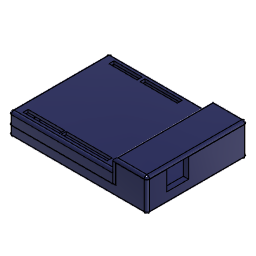
Arduino Case (Autodesk Fusion 360 design; units mm, degrees)
Autodesk Fusion 360 part; units mm, degrees
sketch "Footprint" plane through (0, 0, 0) normal (0, 0, 1) x (1, 0, 0) in component "Box"
  line L0 (-37.3689, 24.9646) -> (33.9311, 24.9646)
  line L1 (33.9311, 24.9646) -> (33.9311, -28.6454)
  line L2 (33.9311, -28.6454) -> (-37.3689, -28.6454)
  line L3 (-39.9289, -28.6454) -> (-39.9289, 24.9646) construction
  line L4 (-37.3689, 24.9646) -> (-37.3689, 23.8242)
  line L5 (-37.3689, -17.1454) -> (-37.3689, -28.6454)
  line L6 (-39.9289, -12.7954) -> (-39.9289, 20.8146)
  line L7 (-37.3689, -28.6454) -> (-39.9289, -28.6454) construction
  line L8 (-37.3689, 24.9646) -> (-39.9289, 24.9646) construction
  spline S0 degree 5 poles (-37.3689, -17.1454) (-37.4677, -17.1053) (-37.6612, -17.0209) (-37.9387, -16.8819) (-38.2829, -16.671) (-38.6672, -16.3623) (-39.0017, -16.0045) (-39.2827, -15.5942) (-39.5091, -15.13) (-39.6839, -14.6151) (-39.8112, -14.0534) (-39.8784, -13.57) (-39.9106, -13.1896) (-39.9241, -12.9281) (-39.9289, -12.7954) knots 0 0 0 0 0 0 0.1 0.2 0.3 0.4 0.5 0.6 0.7 0.8 0.9 1 1 1 1 1 1
  spline S1 degree 5 poles (-37.3689, 23.8242) (-37.4546, 23.8427) (-37.6228, 23.8724) (-37.8658, 23.8956) (-38.1706, 23.8828) (-38.5177, 23.7895) (-38.8283, 23.6128) (-39.1, 23.3478) (-39.3331, 22.9945) (-39.5301, 22.5591) (-39.6944, 22.0491) (-39.802, 21.5868) (-39.8702, 21.2116) (-39.9102, 20.949) (-39.9289, 20.8146) knots 0 0 0 0 0 0 0.1 0.2 0.3 0.4 0.5 0.6 0.7 0.8 0.9 1 1 1 1 1 1
  circle A0 centre (-37.3739, -10.6904) radius 1.395
  circle A1 centre (-37.3739, 17.3996) radius 1.395
  circle A2 centre (14.9261, 22.4096) radius 1.395
  circle A3 centre (13.6061, -26.0904) radius 1.395
  line L9 (33.9311, 24.9646) -> (36.9311, 24.9646)
  line L10 (36.9311, 24.9646) -> (36.9311, -28.6454)
  line L11 (36.9311, -28.6454) -> (33.9311, -28.6454)
  line L12 (36.9311, 24.9646) -> (36.9311, 26.7646)
  line L13 (36.9311, 26.7646) -> (-41.7289, 26.7646)
  line L14 (-41.7289, 26.7646) -> (-41.7289, -30.4454)
  line L15 (-41.7289, -30.4454) -> (36.9311, -30.4454)
  line L16 (36.9311, -30.4454) -> (36.9311, -28.6454)
  line L17 (33.9311, -19.1004) -> (36.9311, -19.1004)
  line L18 (36.9311, -6.6204) -> (33.9311, -6.6204)
  line L19 (19.2711, -30.4454) -> (19.2711, -28.6454)
  line L20 (19.2711, 24.9646) -> (19.2711, 26.7646)
  point P0 (-39.2184, -15.6652)
  point P1 (-38.9763, 23.4524)
  dimension "d4" = 53.61
  dimension "d6" = 73.86
  dimension "d8" = 2.56
  dimension "d10" = 33.61
  dimension "d12" = 15.85
  dimension "d14" = 2.79
  dimension "d15" = 17.955
  dimension "d16" = 2.555
  dimension "d17" = 7.565
  dimension "d18" = 2.555
  dimension "d19" = 2.555
  dimension "d20" = 20.325
  dimension "d21" = 19.005
  dimension "d22" = 3
  dimension "d23" = 1.8
  dimension "d24" = 1.8
  dimension "d25" = 1.8
  dimension "d31" = 9.545
  dimension "d32" = 12.48
  dimension "d38" = 14.66
  dimension "d47" = 11.5
  constraint horizontal L0
  constraint vertical L1
  constraint horizontal L2
  constraint vertical L3
  constraint perpendicular L0 L4
  constraint coincident L3 L6.end
  constraint coincident L3 L6.start
  constraint perpendicular L2 L5
  constraint collinear L4 L5
  constraint perpendicular L3 L7
  constraint perpendicular L3 L8
  constraint equal A0 A1
  constraint vertical A0.centre A1.centre
  constraint equal A0 A3
  constraint equal A0 A2
  constraint perpendicular L1 L9
  constraint perpendicular L2 L10
  constraint perpendicular L1 L11
  constraint perpendicular L9 L12
  constraint perpendicular L12 L13
  constraint perpendicular L13 L14
  constraint perpendicular L10 L15
  constraint perpendicular L11 L16
  constraint coincident L1 L17.start
  constraint coincident L10 L17.end
  constraint perpendicular L10 L17
  constraint coincident L10 L18.start
  constraint coincident L1 L18.end
  constraint perpendicular L1 L18
  constraint coincident L15 L19.start
  constraint coincident L2 L19.end
  constraint perpendicular L2 L19
  constraint coincident L0 L20.start
  constraint coincident L13 L20.end
  constraint perpendicular L13 L20
  constraint collinear L19 L20
  measures "d4" distance of L0 L2
  measures "d6" distance of L1 L3
  measures "d8" distance of L3 L5
  measures "d10" distance of L6.end L6.start
  measures "d12" distance of L2 L6.start
  measures "d14" diameter of A0
  measures "d15" distance of L2 A0.centre
  measures "d16" distance of L3 A0.centre
  measures "d17" distance of L0 A1.centre
  measures "d18" distance of L2 A3.centre
  measures "d19" distance of L0 A2.centre
  measures "d20" distance of L1 A3.centre
  measures "d21" distance of L1 A2.centre
  measures "d22" distance of L1 L10
  measures "d23" distance of L0 L13
  measures "d24" distance of L2 L15
  measures "d25" distance of L6 L14
  measures "d31" distance of L2 L17
  measures "d32" distance of L17 L18
  measures "d38" distance of L1 L19
  measures "d47" distance of L5.start L2.end
extrude "Extrude1" add sketch "Footprint" along normal blind 1.8 contours L0 L2 L4 L5 L6 S0 S1 L13 L14 L15 L19 L20 | L0 L1 L2 L4 L5 L6 S0 S1 | L0 L9 L12 L13 L20 | L1 L9 L10 L18 | L1 L10 L17 L18 | L1 L10 L11 L17 | L2 L11 L15 L16 L19 | A0 | A1 | A2 | A3 makes body 1 in component "Box"
extrude "Extrude2" add sketch "Footprint" along normal blind 4.5 from surface at 1.8 contours L0 L2 L4 L5 L6 S0 S1 L13 L14 L15 L19 L20 | L0 L9 L12 L13 L20 | L1 L9 L10 L18 | L1 L10 L17 L18 | L1 L10 L11 L17 | L2 L11 L15 L16 L19 | A0 | A1 | A2 | A3 bodies 1 in component "Box"
extrude "Extrude3" add sketch "Footprint" along normal blind 11.08 from surface at 6.3 contours L0 L9 L12 L13 L20 | L1 L9 L10 L18 | L1 L10 L11 L17 | L2 L11 L15 L16 L19 bodies 1 in component "Box"
sketch "Side Profile" plane through (0, 26.7646, 0) normal (0, 1, 0) x (-1, 0, 0) in component "FrontCover"
  line L0 (-19.2711, 6.3) -> (-19.2711, 17.38) construction
  line L1 (-36.9311, 17.38) -> (-19.2711, 17.38) construction
  line L2 (-36.9311, 17.535) -> (-19.1161, 17.535)
  line L3 (-19.1161, 17.535) -> (-19.1161, 6.455)
  line L4 (-19.1161, 6.455) -> (-17.5161, 6.455)
  line L5 (-17.5161, 6.455) -> (-17.5161, 19.035)
  line L6 (-17.5161, 19.035) -> (-36.9311, 19.035)
  line L7 (-36.9311, 19.035) -> (-36.9311, 17.535)
  dimension "d39" = 0.155
  dimension "d40" = 0.155
  dimension "d44" = 0.155
  dimension "d45" = 1.5
  dimension "d46" = 1.6
  constraint parallel L1 L2
  constraint perpendicular L2 L3
  constraint perpendicular L3 L4
  constraint perpendicular L4 L5
  constraint perpendicular L5 L6
  constraint perpendicular L2 L7
  constraint collinear L1.start L2.start L6.end
  measures "d39" distance of L1 L2
  measures "d40" distance of L0 L3
  measures "d44" distance of L0.start L4
  measures "d45" distance of L2 L6
  measures "d46" distance of L3 L5
extrude "Extrude1'" add sketch "Side Profile" against normal up to surface (57.21 mm away) separate body makes body 2 in component "FrontCover"
ref_plane "WorkPlane1" through (-11.2289, -1.8404, 11.4) normal (0, 0, 1) x (1, 0, 0) in component "Lid"
sketch "Footprint (2)" plane through (0, 0, 11.4) normal (0, 0, 1) x (-1, 0, 0) in component "Lid"
  line L0 (-33.9311, 28.6454) -> (37.3689, 28.6454) construction
  line L1 (37.3689, 17.1454) -> (37.3689, 28.6454)
  spline S0 degree 5 poles (37.3689, 17.1454) (37.4677, 17.1053) (37.6612, 17.0209) (37.9387, 16.8819) (38.2829, 16.671) (38.6672, 16.3623) (39.0017, 16.0045) (39.2827, 15.5942) (39.5091, 15.13) (39.6839, 14.6151) (39.8112, 14.0534) (39.8784, 13.57) (39.9106, 13.1896) (39.9241, 12.9281) (39.9289, 12.7954) knots 0 0 0 0 0 0 0.1 0.2 0.3 0.4 0.5 0.6 0.7 0.8 0.9 1 1 1 1 1 1
  line L2 (39.9289, 12.7954) -> (39.9289, -20.8146)
  spline S1 degree 5 poles (37.3689, -23.8242) (37.4546, -23.8427) (37.6228, -23.8724) (37.8658, -23.8956) (38.1706, -23.8828) (38.5177, -23.7895) (38.8283, -23.6128) (39.1, -23.3478) (39.3331, -22.9945) (39.5301, -22.5591) (39.6944, -22.0491) (39.802, -21.5868) (39.8702, -21.2116) (39.9102, -20.949) (39.9289, -20.8146) knots 0 0 0 0 0 0 0.1 0.2 0.3 0.4 0.5 0.6 0.7 0.8 0.9 1 1 1 1 1 1
  line L3 (37.3689, -24.9646) -> (37.3689, -23.8242)
  line L4 (37.3689, -24.9646) -> (-33.9311, -24.9646) construction
  line L5 (41.7289, -26.7646) -> (-17.5161, -26.7646)
  line L6 (-17.5161, -26.7646) -> (-17.5161, -24.9646)
  line L7 (37.3689, -24.9646) -> (-17.5161, -24.9646)
  line L8 (37.3689, 28.6454) -> (-17.5161, 28.6454)
  line L9 (-17.5161, 30.4454) -> (-17.5161, 28.6454)
  line L10 (-17.5161, 30.4454) -> (41.7289, 30.4454)
  line L11 (41.7289, 30.4454) -> (41.7289, -26.7646)
  line L12 (-17.5161, -24.9646) -> (-17.5161, 28.6454)
  line L13 (36.6039, 27.4304) -> (-11.3161, 27.4304)
  line L14 (-11.3161, 27.4304) -> (-11.3161, 24.6204)
  line L15 (-11.3161, 24.6204) -> (36.6039, 24.6204)
  line L16 (36.6039, 24.6204) -> (36.6039, 27.4304)
  line L17 (36.0739, -23.7896) -> (-2.8261, -23.7896)
  line L18 (-2.8261, -23.7896) -> (-2.8261, -20.9796)
  line L19 (-2.8261, -20.9796) -> (36.0739, -20.9796)
  line L20 (36.0739, -20.9796) -> (36.0739, -23.7896)
  line L21 (15.7639, 24.6204) -> (15.7639, 27.4304)
  line L22 (14.8339, 24.6204) -> (14.8339, 27.4304)
  line L23 (20.0439, -23.7896) -> (20.0439, -20.9796)
  line L24 (18.3339, -23.7896) -> (18.3339, -20.9796)
  point P0 (41.7289, -26.7646)
  point P1 (-19.2711, -26.7646)
  point P2 (-19.2711, 30.4454)
  point P3 (41.7289, 30.4454)
  dimension "d48" = 1.755
  dimension "d58" = 0.765
  dimension "d59" = 2.81
  dimension "d60" = 20.84
  dimension "d61" = 0.93
  dimension "d62" = 26.15
  dimension "d63" = 1.215
  dimension "d64" = 1.295
  dimension "d65" = 16.03
  dimension "d66" = 1.71
  dimension "d67" = 21.16
  dimension "d68" = 2.81
  dimension "d69" = 1.175
  constraint coincident P0 L5.start
  constraint horizontal L5
  constraint coincident L4 L6.end
  constraint perpendicular L4 L6
  constraint coincident L3.start L4.start
  constraint coincident L0.end L1.end
  constraint coincident L0 L8.end
  constraint perpendicular L8 L9
  constraint coincident P3 L10.end
  constraint perpendicular L9 L10
  constraint collinear L6 L9
  constraint horizontal L13
  constraint vertical L14
  constraint horizontal L15
  constraint vertical L16
  constraint horizontal L17
  constraint vertical L18
  constraint horizontal L19
  constraint vertical L20
  constraint coincident L15 L21.start
  constraint coincident L13 L21.end
  constraint perpendicular L13 L21
  constraint coincident L15 L22.start
  constraint coincident L13 L22.end
  constraint perpendicular L13 L22
  constraint coincident L17 L23.start
  constraint coincident L19 L23.end
  constraint perpendicular L19 L23
  constraint coincident L17 L24.start
  constraint coincident L19 L24.end
  constraint perpendicular L19 L24
  measures "d48" distance of P1 L6
  measures "d58" distance of L1 L16
  measures "d59" distance of L13 L15
  measures "d60" distance of L16 L21
  measures "d61" distance of L21 L22
  measures "d62" distance of L14 L22
  measures "d63" distance of L8 L13
  measures "d64" distance of S1.start L20
  measures "d65" distance of L20 L23
  measures "d66" distance of L23 L24
  measures "d67" distance of L18 L24
  measures "d68" distance of L17 L19
  measures "d69" distance of L4 L17
extrude "Extrude1''" add sketch "Footprint (2)" along normal blind 1.6 separate body contours L1 S0 L2 S1 L3 L7 L8 L12 | L1 S0 L2 S1 L3 L5 L6 L7 L8 L9 L10 L11 | L13 L15 L21 L22 | L17 L19 L23 L24 makes body 3 in component "Lid"
extrude "Extrude2'" add sketch "Footprint (2)" against normal up to surface (5.255 mm away) contours L1 S0 L2 S1 L3 L5 L6 L7 L8 L9 L10 L11 bodies 3 in component "Lid"
fillet "Fillet1" radius 1.5 4 edges at (-41.7289, 26.7646, 3.15) (36.9311, 26.7646, 8.69) (36.9311, -30.4454, 8.69) (-41.7289, -30.4454, 3.15) 1 faces at (-15.5089, 7.6946, 0) on bodies 1 in component "Box"
fillet "Fillet1'" radius 1.5 6 edges at (27.2236, 26.7646, 19.035) (36.9311, 26.7646, 18.285) (27.2236, -30.4454, 19.035) (36.9311, -30.4454, 18.285) (17.5161, -1.8404, 19.035) (36.9311, -1.8404, 19.035) on bodies 2 in component "FrontCover"
fillet "Fillet1''" radius 1.5 5 edges at (-41.7289, 26.7646, 9.5725) (-41.7289, -30.4454, 9.5725) (-41.7289, -1.8404, 13) (-12.1064, -30.4454, 13) (-12.1064, 26.7646, 13) on bodies 3 in component "Lid"
component "Box" placed x (1, 0, 0) y (0, 1, 0) z (0, 0, 1) at (0, 0, 0)
component "FrontCover" placed x (1, 0, 0) y (0, 1, 0) z (0, 0, 1) at (0, 0, 0)
component "Lid" placed x (1, 0, 0) y (0, 1, 0) z (0, 0, 1) at (0, 0, 0)
equation "Tolerance = 0.17 mm" comment "Tolerance to use when PLA/PETG parts mate with existing parts (like a a screw), or when you a very small amount of clearance at mating site."
equation "Tolerance_Tight = 0.155 mm" comment "Tolerance to use when you want the parts to make contact at mating site."
equation "Tolerance_PressFitLight = 0.12 mm" comment "Tolerance to use when you want the parts to press fit together, like Legos."
equation "d4 = Arduino_Width + 2 * Tolerance_Tight"
equation "Arduino_Width = 53.3 mm"
equation "d6 = Arduino_Length + 2 * Tolerance_Tight"
equation "Arduino_Length = 73.55 mm"
equation "d10 = Arduino_BackBumpLength + 2 * Tolerance_Tight"
equation "Arduino_BackBumpLength = 33.3 mm"
equation "Arduino_MountingHoleDiameter = 3.1 mm"
equation "d14 = Arduino_MountingHoleDiameter - 2 * Tolerance_Tight"
equation "d15 = 2 * Tolerance_Tight + d14 / 2 + 16.25 mm"
equation "d16 = 0.85 mm + d14 / 2 + 2 * Tolerance_Tight"
equation "d17 = 2 * Tolerance_Tight + 5.86 mm + d14 / 2"
equation "d18 = d16"
equation "d19 = d16"
equation "d20 = 2 * Tolerance_Tight + 18.62 mm + d14 / 2"
equation "d21 = 2 * Tolerance_Tight + 17.3 mm + d14 / 2"
equation "d24 = d23"
equation "d25 = d23"
equation "d26 = d23"
equation "d31 = 9.7 mm - Tolerance_Tight"
equation "d32 = Arduino_UsbPortWidth + 2 * Tolerance_Tight"
equation "Arduino_UsbPortHeight = 10.77 mm"
equation "Arduino_UsbPortWidth = 12.17 mm"
equation "d36 = Arduino_UsbPortHeight + 2 * Tolerance_Tight"
equation "d39 = Tolerance_Tight"
equation "d40 = d39"
equation "d44 = d39"
equation "d48 = d46 + Tolerance_Tight"
equation "Arduino_LidHeight = 5.1 mm"
equation "d50 = Arduino_LidHeight"
equation "d53 = -Tolerance_Tight"
equation "d55 = 1.5 mm"
equation "d56 = d55"
equation "d57 = d55"
equation "d58 = 0.92 mm - Tolerance_Tight"
equation "d59 = 2.5 mm + 2 * Tolerance_Tight"
equation "d60 = 20.53 mm + 2 * Tolerance_Tight"
equation "d61 = 1.24 mm - 2 * Tolerance_Tight"
equation "d62 = 25.84 mm + 2 * Tolerance_Tight"
equation "d63 = 1.37 mm - Tolerance_Tight"
equation "d64 = 1.45 mm - Tolerance_Tight"
equation "d65 = 15.72 mm + 2 * Tolerance_Tight"
equation "d66 = 2.02 mm - 2 * Tolerance_Tight"
equation "d67 = 20.85 mm + 2 * Tolerance_Tight"
equation "d68 = d59"
equation "d69 = 1.33 mm - Tolerance_Tight"
